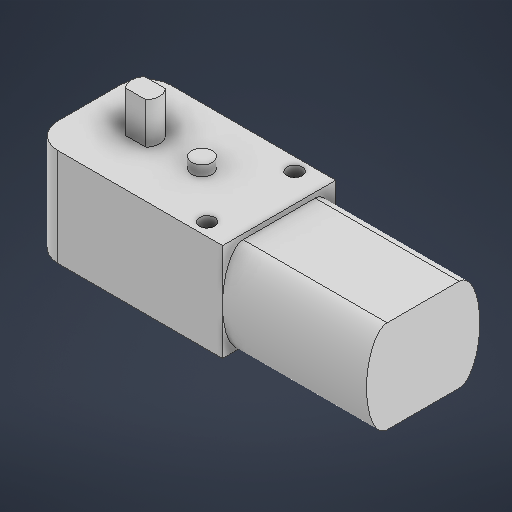
# Autodesk Inventor part: 黄モーター
Saved by Autodesk Inventor 2026 (Build 300175000, 175)
## iProperties
Created: 2025-10-25
Part Number: 黄モーター
Material: 一般
Document SubType Name: Modeling
Designer: masak
Density: 1 g/cm^3
Appearance: 既定
Author: masak
Autodesk Inventor part; units mm, degrees
ref_plane "YZ Plane" through (0, 0, 0) normal (1, 0, 0) x (0, 1, 0)
ref_plane "XZ Plane" through (0, 0, 0) normal (0, 1, 0) x (-1, 0, 0)
ref_plane "XY Plane" through (0, 0, 0) normal (0, 0, 1) x (1, 0, 0)
sketch "スケッチ1" plane through (0, 0, 0) normal (0, 1, 0) x (-1, 0, 0)
  line L0 (0, 0) -> (37, 0)
  line L1 (37, 0) -> (37, -22)
  line L2 (37, -22) -> (0, -22)
  line L3 (0, -22) -> (0, 0)
  line L4 (37, 0) -> (37, -3.6217)
  line L5 (37, 0) -> (32, 0)
  line L6 (32, 0) -> (32, -5)
  line L7 (32, -5) -> (37, -5)
  line L8 (37, -5) -> (37, 0)
  circle A0 centre (32, -5) radius 5
  line L9 (37, -22) -> (32, -22)
  line L10 (32, -22) -> (32, -17)
  line L11 (32, -17) -> (37, -17)
  line L12 (37, -17) -> (37, -22)
  circle A1 centre (32, -17) radius 5
  dimension "d1" = 22
  dimension "d2" = 37
  dimension "d6" = 5
  dimension "d7" = 5
  constraints: 26 end point, 6 parallel, 3 horizontal, 3 perpendicular, 2 coincident, 1 point on line, 6 other
  measures "d1" distance of L2.end L0.start
  measures "d2" distance of L0.start L0.end
  measures "d6" distance of L5.end L6.end
  measures "d7" distance of L9.end L10.end
extrude "押し出し1" add sketch "スケッチ1" along normal blind 19 contours L0 A0 L1 A1 L2 L3 | A0 L7 L6 | L6 L7 A0 | A1 L11 L10 | L10 L11 A1
sketch "スケッチ2" plane through (0, 19, 0) normal (0, 1, 0) x (1, 0, 0)
  line L0 (0, 0) -> (0, 22) projected
  line L1 (0, 0) -> (0, 22)
  line L2 (0, 11) -> (-37, 11)
  line L3 (-37, 17) -> (-37, 5) projected
  line L4 (-37, 11) -> (-26, 11)
  circle A0 centre (-26, 11) radius 2.75
  line L5 (-28, 9.1125) -> (-24, 9.1125)
  line L6 (-28, 12.8875) -> (-24, 12.8875)
  dimension "d10" = 11
  dimension "d11" = 5.5
  dimension "d12" = 4
  constraints: 10 end point, 4 point on circle, 3 midpoint, 1 centre point, 1 coincident, 1 collinear, 1 horizontal, 1 parallel, 1 point on line
  measures "d10" distance of point (-37, 11) L4.end
  measures "d11" diameter of A0
  measures "d12" distance of L5.start L5.end
extrude "押し出し2" add sketch "スケッチ2" along normal blind 8 contours A0 L5 L2 | L2 A0 L6
sketch "スケッチ3" plane through (0, 0, 0) normal (0, -1, 0) x (1, 0, 0)
  arc A0 (-24, -12.8875) -> (-24, -9.1125) centre (-26, -11) ccw projected
  line L0 (-28, -12.8875) -> (-24, -12.8875) projected
  arc A1 (-28, -9.1125) -> (-28, -12.8875) centre (-26, -11) ccw projected
  line L1 (-24, -9.1125) -> (-28, -9.1125) projected
  point P0 (0, 0)
extrude "押し出し3" add sketch "スケッチ3" along normal blind 8
sketch "スケッチ4" plane through (0, 19, 0) normal (0, 1, 0) x (1, 0, 0)
  line L0 (0, 0) -> (0, 22) projected
  line L1 (0, 11) -> (-15, 11)
  circle A0 centre (-15, 11) radius 2
  dimension "d17" = 15
  dimension "d18" = 4
  constraints: 2 end point, 1 centre point, 1 coincident, 1 horizontal, 1 midpoint
  measures "d17" distance of L1.start L1.end
  measures "d18" diameter of A0
extrude "押し出し4" add sketch "スケッチ4" along normal blind 2
sketch "スケッチ5" plane through (0, 0, 0) normal (1, 0, 0) x (0, 0, -1)
  line L0 (22, 0) -> (22, 19) projected
  line L1 (0, 0) -> (22, 0)
  line L2 (22, 0) -> (22, 18)
  line L3 (22, 18) -> (0, 18)
  line L4 (0, 18) -> (0, 0)
  line L5 (0, 0) -> (0, 19) projected
  line L6 (0, 9) -> (22, 9)
  line L7 (11, 0) -> (11, 18)
  line L8 (4, 9) -> (4, 0)
  ellipse E0 centre (4, 9) end of major axis (0, 9) minor radius 9
  ellipse E1 centre (18, 9) end of major axis (22, 9) minor radius 9
  point P0 (4, 18)
  point P1 (18, 0)
  point P2 (18, 18)
  dimension "d21" = 18
  constraints: 14 end point, 4 point on line, 3 midpoint, 2 horizontal, 2 parallel, 2 perpendicular, 1 coincident, 1 symmetric about line, 1 vertical, 6 other
  measures "d21" distance of L3.end L1.start
extrude "押し出し5" add sketch "スケッチ5" along normal blind 28 contours E1 L6 | L6 E1 | L1 L7 L6 E1 | L6 L7 L3 E1 | L1 E0 L6 L7 | L6 E0 L3 L7 | E0 L6 L8 | L8 L6 E0 | L6 E0
sketch "スケッチ6" plane through (0, 19, 0) normal (0, 1, 0) x (1, 0, 0)
  arc A0 (-32, 22) -> (-37, 17) centre (-32, 17) ccw projected
  line L0 (0, 0) -> (0, 22) projected
  line L1 (-32, 22) -> (0, 22)
  line L2 (0, 22) -> (-2.4665, 22)
  line L3 (0, 0) -> (-5.5, 0)
  line L4 (-32, 0) -> (0, 0) projected
  line L5 (-5.5, 0) -> (-5.5, 2.5)
  circle A1 centre (-5.5, 2.5) radius 1.5
  line L6 (0, 11) -> (-37, 11)
  line L7 (-37, 17) -> (-37, 5) projected
  circle A2 centre (-5.5, 19.5) radius 1.5
  dimension "d25" = 5.5
  dimension "d26" = 2.5
  dimension "d27" = 3
  constraints: 10 end point, 2 centre point, 2 midpoint, 2 perpendicular, 2 point on line, 1 coincident, 1 symmetric about line, 1 other
  measures "d25" distance of L0.start L3.end
  measures "d26" distance of L3.end L5.end
  measures "d27" diameter of A1
extrude "押し出し6" cut sketch "スケッチ6" against normal blind 22 contours A1 | A2
